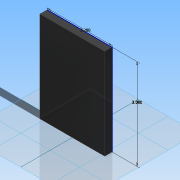
# Autodesk Inventor part: Generic Riser
Saved by Autodesk Inventor 2014 SP2 (Build 180246200, 246)
## iProperties
Created: 2014-05-18
Part Number: Generic Riser
Material: Rubber
Document SubType Name: Modeling
Designer: dliu
Density: 0.93 g/cm^3
Appearance: Rubber - Black - Version 1.1
Author: dliu
Autodesk Inventor part; units mm, degrees
ref_plane "YZ Plane" through (0, 0, 0) normal (1, 0, 0) x (0, 1, 0)
ref_plane "XZ Plane" through (0, 0, 0) normal (0, 1, 0) x (-1, 0, 0)
ref_plane "XY Plane" through (0, 0, 0) normal (0, 0, 1) x (1, 0, 0)
sketch "Sketch1" plane through (0, 0, 0) normal (0, 0, 1) x (1, 0, 0)
  line L0 (-27.94, 39.116) -> (27.94, 39.116)
  line L1 (27.94, 39.116) -> (27.94, -39.116)
  line L2 (27.94, -39.116) -> (-27.94, -39.116)
  line L3 (-27.94, -39.116) -> (-27.94, 39.116)
  line L4 (-27.94, 39.116) -> (27.94, -39.116) construction
  line L5 (27.94, 39.116) -> (-27.94, -39.116) construction
  point P0 (0, 0)
  dimension "d2" = 55.88
  dimension "d3" = 78.232
  constraints: 12 end point, 2 midpoint, 2 parallel, 1 horizontal, 1 perpendicular
  measures "d2" distance of L0.start L0.end
  measures "d3" distance of L0.end L1.end
extrude "Extrusion1" add sketch "Sketch1" along normal blind 6.35
body "Solid1"
